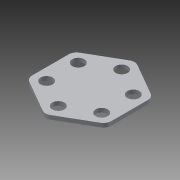
# Autodesk Inventor part: Roller Pneumatic Back Connector (Custom)
Saved by Autodesk Inventor 2014 (Build 180170000, 170)
## iProperties
Created: 2014-01-06
Part Number: Roller Pneumatic Back Connector (Custom)
Material: Aluminum 6061
Document SubType Name: Modeling
Designer: Andrew Toennies
Density: 2.71 g/cm^3
Appearance: Aluminum - Flat
Mass: 3.30976 g
Surface Area: 18.4784 cm^2
Volume: 1.22131 cm^3
Author: Andrew Toennies
Autodesk Inventor part; units mm, degrees
ref_plane "YZ Plane" through (0, 0, 0) normal (1, 0, 0) x (0, 1, 0)
ref_plane "XZ Plane" through (0, 0, 0) normal (0, 1, 0) x (-1, 0, 0)
ref_plane "XY Plane" through (0, 0, 0) normal (0, 0, 1) x (1, 0, 0)
sketch "Sketch1" plane through (0, 0, 0) normal (0, 1, 0) x (-1, 0, 0)
  circle A0 centre (0, 0) radius 2.413
  circle A1 centre (0, 25.4) radius 2.413
  line L0 (0, 25.4) -> (0, 0) construction
  circle A2 centre (11.049, 19.05) radius 2.413
  circle A3 centre (11.049, 6.35) radius 2.413
  circle A4 centre (-11.049, 6.35) radius 2.413
  circle A5 centre (-11.049, 19.05) radius 2.413
  line L1 (-11.049, 6.35) -> (-11.049, 19.05) construction
  line L2 (-11.049, 19.05) -> (11.049, 19.05) construction
  line L3 (1.5875, 30.1143) -> (14.2875, 22.782)
  line L4 (15.875, 20.0323) -> (15.875, 5.3677)
  line L5 (14.2875, 2.618) -> (1.5875, -4.7143)
  line L6 (-1.5875, -4.7143) -> (-14.2875, 2.618)
  line L7 (-15.875, 5.3677) -> (-15.875, 20.0323)
  line L8 (-14.2875, 22.782) -> (-1.5875, 30.1143)
  arc A6 (1.5875, 30.1143) -> (-1.5875, 30.1143) centre (0, 27.3647) ccw
  arc A7 (-14.2875, 22.782) -> (-15.875, 20.0323) centre (-12.7, 20.0323) ccw
  arc A8 (-15.875, 5.3677) -> (-14.2875, 2.618) centre (-12.7, 5.3677) ccw
  arc A9 (-1.5875, -4.7143) -> (1.5875, -4.7143) centre (0, -1.9647) ccw
  arc A10 (14.2875, 2.618) -> (15.875, 5.3677) centre (12.7, 5.3677) ccw
  arc A11 (15.875, 20.0323) -> (14.2875, 22.782) centre (12.7, 20.0323) ccw
  point P0 (0, 12.7)
  point P1 (0, 31.0309)
  point P2 (15.875, 21.8654)
  point P3 (15.875, 3.5346)
  point P4 (0, -5.6309)
  point P5 (-15.875, 3.5346)
  point P6 (-15.875, 21.8654)
  dimension "d1" = 4.826
  dimension "d2" = 25.4
  dimension "d3" = 4.826
  dimension "d4" = 4.826
  dimension "d5" = 12.7
  dimension "d6" = 11.049
  dimension "d7" = 11.049
  dimension "d8" = 6.35
  dimension "d9" = 4.826
  dimension "d10" = 4.826
  dimension "d11" = 11.049
  dimension "d12" = 12.7
  dimension "d13" = 31.75
  dimension "d14" = 3.175
  constraints: 18 end point, 13 point on line, 12 centre point, 12 point on circle, 12 tangent, 6 equal radius, 1 coincident, 1 midpoint, 1 parallel, 1 perpendicular, 1 vertical, 13 other
  measures "d1" diameter of A1
  measures "d2" distance of L0.start L0.end
  measures "d3" diameter of A2
  measures "d4" diameter of A3
  measures "d5" distance of A3.centre L2.end
  measures "d6" distance from line of L0 A3.centre
  measures "d7" distance from line of L0 L2.end
  measures "d8" vertical distance of point (0, 0) A3.centre
  measures "d9" diameter of A4
  measures "d10" diameter of A5
  measures "d11" distance between parallel lines of L1 L0
  measures "d12" distance of L1.start L1.end
  measures "d13" distance between parallel lines of L7 L4
  measures "d14" radius of A6
extrude "Extrusion1" add sketch "Sketch1" along normal blind 1.5875
body "Solid1"
